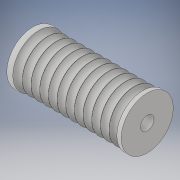
# Autodesk Inventor part: Polycord conveyor2
Saved by Autodesk Inventor 2018 (Build 220112000, 112)
## iProperties
Created: 2020-02-05
Part Number: Polycord conveyor2
Material: Generic
Document SubType Name: Modeling
Designer: Burni
Density: 1 g/cm^3
Appearance: Default
Author: Burni
Autodesk Inventor part; units mm, degrees
ref_plane "YZ Plane" through (0, 0, 0) normal (1, 0, 0) x (0, 1, 0)
ref_plane "XZ Plane" through (0, 0, 0) normal (0, 1, 0) x (-1, 0, 0)
ref_plane "XY Plane" through (0, 0, 0) normal (0, 0, 1) x (1, 0, 0)
sketch "Sketch1" plane through (0, 0, 0) normal (0, 0, 1) x (1, 0, 0)
  line L0 (-11.4113, -1.4037) -> (-95.2313, -1.4037)
  line L1 (-95.2313, -1.4037) -> (-95.2313, 17.6463)
  line L2 (-11.4113, 17.6463) -> (-11.4113, -1.4037)
  line L3 (-11.4113, 17.6463) -> (-14.5863, 17.6463)
  arc A0 (-20.9363, 17.6463) -> (-14.5863, 17.6463) centre (-17.7613, 17.6463) ccw
  arc A1 (-27.2863, 17.6463) -> (-20.9363, 17.6463) centre (-24.1113, 17.6463) ccw
  arc A2 (-33.6363, 17.6463) -> (-27.2863, 17.6463) centre (-30.4613, 17.6463) ccw
  arc A3 (-39.9863, 17.6463) -> (-33.6363, 17.6463) centre (-36.8113, 17.6463) ccw
  arc A4 (-46.3363, 17.6463) -> (-39.9863, 17.6463) centre (-43.1613, 17.6463) ccw
  arc A5 (-52.6863, 17.6463) -> (-46.3363, 17.6463) centre (-49.5113, 17.6463) ccw
  arc A6 (-59.0363, 17.6463) -> (-52.6863, 17.6463) centre (-55.8613, 17.6463) ccw
  line L4 (-95.2313, 17.6463) -> (-90.7863, 17.6463)
  arc A7 (-65.3863, 17.6463) -> (-59.0363, 17.6463) centre (-62.2113, 17.6463) ccw
  arc A8 (-90.7863, 17.6463) -> (-84.4363, 17.6463) centre (-87.6113, 17.6463) ccw
  line L5 (-11.4113, -1.4037) -> (-95.2313, -1.4037)
  line L6 (-95.2313, -1.4037) -> (-95.2313, 3.5493)
  line L7 (-95.2313, 3.5493) -> (-11.4113, 3.5493)
  line L8 (-11.4113, 3.5493) -> (-11.4113, -1.4037)
  line L9 (-11.4113, -1.4037) -> (-11.4113, 3.5493)
  line L10 (-95.2313, -1.4037) -> (-95.2313, 3.5493)
  line L11 (-11.4113, 3.5493) -> (-95.2313, 3.5493)
  line L12 (-95.2313, -1.4037) -> (-11.4113, -1.4037)
  arc A9 (-71.7363, 17.6463) -> (-65.3863, 17.6463) centre (-68.5613, 17.6463) ccw
  arc A10 (-78.0863, 17.6463) -> (-71.7363, 17.6463) centre (-74.9113, 17.6463) ccw
  arc A11 (-84.4363, 17.6463) -> (-78.0863, 17.6463) centre (-81.2613, 17.6463) ccw
  line L13 (-11.4113, 17.6463) -> (-11.4113, 3.5493)
  line L14 (-95.2313, 3.5493) -> (-95.2313, 17.6463)
  line L15 (-95.2313, 17.6463) -> (-90.7863, 17.6463)
  line L16 (-90.7863, 17.6463) -> (-90.7863, 17.0113)
  line L17 (-90.7863, 17.0113) -> (-14.5863, 17.0113) construction
  line L18 (-14.5863, 17.0113) -> (-14.5863, 17.6463)
  line L19 (-11.4113, 14.4713) -> (-11.4113, 17.0113)
  line L20 (-95.2313, 17.0113) -> (-95.2313, 14.4713)
  line L21 (-84.5005, 17.0113) -> (-84.3722, 17.0113)
  line L22 (-78.1505, 17.0113) -> (-78.0222, 17.0113)
  line L23 (-71.8005, 17.0113) -> (-71.6722, 17.0113)
  line L24 (-65.4505, 17.0113) -> (-65.3222, 17.0113)
  line L25 (-59.1005, 17.0113) -> (-58.9722, 17.0113)
  line L26 (-52.7505, 17.0113) -> (-52.6222, 17.0113)
  line L27 (-46.4005, 17.0113) -> (-46.2722, 17.0113)
  line L28 (-40.0505, 17.0113) -> (-39.9222, 17.0113)
  line L29 (-33.7005, 17.0113) -> (-33.5722, 17.0113)
  line L30 (-27.3505, 17.0113) -> (-27.2222, 17.0113)
  line L31 (-21.0005, 17.0113) -> (-20.8722, 17.0113)
  dimension "d33" = 19.05
  dimension "d34" = 83.82
  dimension "d35" = 3.175
  dimension "d40" = 3.175
  dimension "d43" = 3.175
  dimension "d44" = 3.175
  dimension "d46" = 3.175
  dimension "d47" = 3.175
  dimension "d56" = 3.175
  dimension "d59" = 3.175
  dimension "d60" = 90
  dimension "d63" = 3.175
  dimension "d70" = 3.175
  dimension "d71" = 0
  dimension "d72" = 4.953
  dimension "d73" = 3.175
  dimension "d75" = 3.175
  dimension "d76" = 3.175
  dimension "d77" = 0.635
  dimension "d78" = 4.445
  dimension "d79" = 90
  constraints: 62 end point, 47 point on circle, 12 centre point, 4 collinear, 4 parallel, 4 tangent, 4 vertical, 3 horizontal, 3 point on line, 2 perpendicular, 25 other
  measures "d33" distance of L0.end L1.end
  measures "d34" distance of L0.start L0.end
  measures "d35" distance of L2.start L3.end
  measures "d40" radius of A0
  measures "d43" radius of A1
  measures "d44" radius of A2
  measures "d46" radius of A3
  measures "d47" radius of A4
  measures "d56" radius of A5
  measures "d59" radius of A6
  measures "d60" angle of L2 L3
  measures "d63" radius of A7
  measures "d70" radius of A8
  measures "d71" distance of A8.start L4.end
  measures "d72" distance of L7.end L0.start
  measures "d73" radius of A9
  measures "d75" radius of A10
  measures "d76" radius of A11
  measures "d77" distance of L15.end L16.end
  measures "d78" distance of L1.end L4.end
  measures "d79" angle of L1 L4
revolve "Revolution3" add sketch "Sketch1" angle 360 about axis through (-11.4113, -1.4037, 0) along (-1, 0, 0) contours L7 L1 L4 A8 L21 A11 L22 A10 L23 A9 L24 A7 L25 A6 L26 A5 L27 A4 L28 A3 L29 A2 L30 A1 L31 A0 L3 L2
equation "\"d43\" = d40"
equation "\"d44\" = d40"
equation "\"d46\" = d40"
equation "\"d47\" = d46"
equation "\"d56\" = d40"
equation "\"d59\" = d40"
equation "\"d63\" = d40"
equation "\"d73\" = d40"
equation "\"d75\" = d73"
equation "\"d76\" = d75"
body "Solid3"
